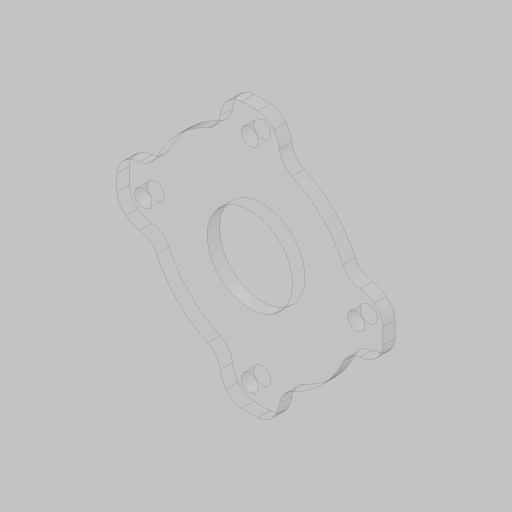
# Autodesk Inventor part: CL7-020
Saved by Autodesk Inventor 2023.5 (Build 275446000, 446)
## iProperties
Created: 2025-03-18
Part Number: CL7-020
Material: Polycarbonate, Clear
Document SubType Name: Modeling
Designer: brand
Density: 1.2 g/cm^3
Appearance: Polycarbonate - Clear
Author: brand
Autodesk Inventor part; units mm, degrees
ref_plane "YZ Plane" through (0, 0, 0) normal (1, 0, 0) x (0, 1, 0)
ref_plane "XZ Plane" through (0, 0, 0) normal (0, 1, 0) x (-1, 0, 0)
ref_plane "XY Plane" through (0, 0, 0) normal (0, 0, 1) x (1, 0, 0)
sketch "Sketch1" plane through (0, 0, 0) normal (0, 0, 1) x (1, 0, 0)
  circle A0 centre (0, 0) radius 23.8125
  circle A1 centre (0, 0) radius 39.6875
  circle A2 centre (0, 0) radius 31.75 construction
  circle A3 centre (0, 0) radius 12.7
  point P0 (0, 31.75)
  point P1 (-31.75, 0)
  point P2 (31.75, 0)
  point P3 (0, -31.75)
  dimension "d0" = 47.625
  dimension "d1" = 15.875
  dimension "d2" = 63.5
  dimension "d5" = 25.4
  constraints: 4 centre point, 4 point on circle, 3 coincident, 2 horizontal alignment, 2 vertical alignment
  measures "d0" diameter of A0
  measures "d1" radial gap between concentric circles of A0 A1
  measures "d2" diameter of A2
  measures "d5" diameter of A3
extrude "Extrusion1" add sketch "Sketch1" against normal blind 3.683 contours A0 | A1
extrude "Extrusion2" [suppressed]
hole "Hole1" at (0, 31.75, 0) at (-31.75, 0, 0) at (31.75, 0, 0) at (0, -31.75, 0) direction (0, 0, -1) diameter 5.1054 end through all clearance for "Flat Head Machine Screw (82)" size "#10" standard "Ansi Unified Screw Threads"
sketch "Sketch2" plane through (0, 0, 0) normal (0, 0, 1) x (1, 0, 0)
  circle A0 centre (31.75, 0) radius 2.5527 construction
  circle A1 centre (0, 31.75) radius 2.5527 construction
  circle A2 centre (-31.75, 0) radius 2.5527 construction
  circle A3 centre (0, -31.75) radius 2.5527 construction
  circle A4 centre (0, 0) radius 39.6875 construction
  circle A5 centre (0, 31.75) radius 8.9027 construction
  circle A6 centre (31.75, 0) radius 8.9027 construction
  circle A7 centre (0, 0) radius 30.454 construction
  circle A8 centre (-31.75, 0) radius 8.9027 construction
  circle A9 centre (0, -31.75) radius 8.9027 construction
  arc A10 (-27.7553, -12.5336) -> (-32.7963, -8.841) centre (-33.5426, -15.147) ccw
  line L0 (0, 0) -> (-28.0633, -28.0633) construction
  line L1 (0, 0) -> (-31.75, 0) construction
  circle A11 centre (0, 0) radius 39.6875 construction
  arc A12 (-39.4315, -4.5002) -> (-32.7963, -8.841) centre (-31.75, 0) ccw
  arc A13 (-27.7553, -12.5336) -> (-12.5336, -27.7553) centre (0, 0) ccw
  arc A14 (-8.841, -32.7963) -> (-12.5336, -27.7553) centre (-15.147, -33.5426) ccw
  line L2 (-33.5426, -15.147) -> (-15.147, -33.5426) construction
  circle A15 centre (-31.75, 0) radius 2.5527 construction
  line L3 (0, 0) -> (-31.75, 0) construction
  line L4 (0, 0) -> (0, -31.75) construction
  arc A16 (-8.841, -32.7963) -> (-4.5002, -39.4315) centre (0, -31.75) ccw
  arc A17 (-32.7963, 8.841) -> (-27.7553, 12.5336) centre (-33.5426, 15.147) ccw
  arc A18 (-32.7963, 8.841) -> (-39.4315, 4.5002) centre (-31.75, 0) ccw
  arc A19 (-12.5336, 27.7553) -> (-27.7553, 12.5336) centre (0, 0) ccw
  arc A20 (-12.5336, 27.7553) -> (-8.841, 32.7963) centre (-15.147, 33.5426) ccw
  arc A21 (-4.5002, 39.4315) -> (-8.841, 32.7963) centre (0, 31.75) ccw
  arc A22 (-39.4315, 4.5002) -> (-39.4315, -4.5002) centre (0, 0) ccw construction
  line L5 (0, 0) -> (28.0633, -28.0633) construction
  circle A23 centre (0, 0) radius 39.6875 construction
  circle A24 centre (0, 0) radius 39.6875
  arc A25 (32.7963, -8.841) -> (27.7553, -12.5336) centre (33.5426, -15.147) ccw
  arc A26 (18.6424, -24.0812) -> (27.7553, -12.5336) centre (0, 0) ccw
  arc A27 (4.5002, -39.4315) -> (7.4557, -36.6153) centre (0, -31.75) ccw
  arc A28 (32.7963, -8.841) -> (39.4315, -4.5002) centre (31.75, 0) ccw
  circle A29 centre (0, 0) radius 12.7 projected
  point P0 (-4.5002, 39.4315)
  point P1 (-39.4315, 4.5002)
  point P2 (-39.4315, -4.5002)
  point P3 (-4.5002, -39.4315)
  dimension "d15" = 6.35
  dimension "d16" = 6.35
  dimension "d18" = 6.35
  dimension "d19" = 6.35
  dimension "d20" = 45
  dimension "d21" = 6.35
  dimension "d22" = 45
  dimension "d27" = 6.35
  constraints: 42 point on circle, 20 centre point, 14 symmetric about line, 12 end point, 7 coincident, 5 tangent, 3 concentric, 2 horizontal, 2 point on line, 1 vertical, 13 other
  measures "d15" radial gap between concentric circles of A1 A5
  measures "d16" radial gap between concentric circles of A0 A6
  measures "d18" radial gap between concentric circles of A2 A8
  measures "d19" radial gap between concentric circles of A3 A9
  measures "d20" angle of L0 L1
  measures "d21" radius of A10
  measures "d22" angle of L5 L4
  measures "d27" radius of A25
extrude "Extrusion3" cut sketch "Sketch2" against normal through all contours A13 A14 A16 A24 A12 A10 | A24 A21 A20 A19 A17 A18
mirror "Mirror1" about plane through (0, 0, 0) normal (1, 0, 0) of "Extrusion3"
fillet "Fillet1" radius 6.35 8 edges at (-39.4315, 4.5002, -1.8415) (-39.4315, -4.5002, -1.8415) (4.5002, 39.4315, -1.8415) (-4.5002, 39.4315, -1.8415) (39.4315, 4.5002, -1.8415) (39.4315, -4.5002, -1.8415) (4.5002, -39.4315, -1.8415) (-4.5002, -39.4315, -1.8415)
equation "\"d22\" = d20"
equation "\"d27\" = d26"
equation "\"d26\" = d21"
body "Solid1"
